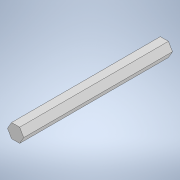
# Autodesk Inventor part: P88042_Wheel_Hex_Pin_B
Saved by Autodesk Inventor 2022.3 (Build 263350000, 350)
## iProperties
Created: 2022-07-07
Part Number: P88042_Wheel_Hex_Pin_B
Material: Generic
Document SubType Name: Modeling
Designer: luis_
Density: 1 g/cm^3
Appearance: Default
Author: luis_
Autodesk Inventor part; units mm, degrees
ref_plane "YZ Plane" through (0, 0, 0) normal (1, 0, 0) x (0, 1, 0)
ref_plane "XZ Plane" through (0, 0, 0) normal (0, 1, 0) x (-1, 0, 0)
ref_plane "XY Plane" through (0, 0, 0) normal (0, 0, 1) x (1, 0, 0)
extrude "Extrusion1" [suppressed]
sketch "Sketch2" plane through (0, 0, 0) normal (0, 0, 1) x (1, 0, 0)
  line L0 (1.4434, 0) -> (0.7217, -1.25)
  line L1 (0.7217, -1.25) -> (-0.7217, -1.25)
  line L2 (-0.7217, -1.25) -> (-1.4434, 0)
  line L3 (-1.4434, 0) -> (-0.7217, 1.25)
  line L4 (-0.7217, 1.25) -> (0.7217, 1.25)
  line L5 (0.7217, 1.25) -> (1.4434, 0)
  point P0 (0, 0)
  point P1 (0, 0)
  point P2 (0, 1.25)
  dimension "d6" = 1.25
  constraints: 12 end point, 1 coincident, 1 midpoint, 13 other
  measures "d6" distance of point (0, 1.25) point (0, 0)
extrude "Extrusion2" add sketch "Sketch2" against normal blind 26.5
body "Solid1"
